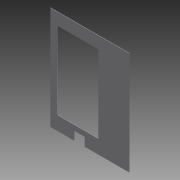
# Autodesk Inventor part: Right Side
Saved by Autodesk Inventor 2012 (Build 160160000, 160)
## iProperties
Created: 2012-04-20
Part Number: Right Side
Material: Default
Document SubType Name: Modeling
Designer: Puzzles
Density: 1 g/cm^3
Author: Puzzles
Autodesk Inventor part; units mm, degrees
ref_plane "YZ Plane" through (0, 0, 0) normal (1, 0, 0) x (0, 1, 0)
ref_plane "XZ Plane" through (0, 0, 0) normal (0, 1, 0) x (-1, 0, 0)
ref_plane "XY Plane" through (0, 0, 0) normal (0, 0, 1) x (1, 0, 0)
sketch "Sketch1" plane through (0, 0, 0) normal (0, 0, 1) x (1, 0, 0)
  line L0 (-292.1, 381) -> (292.1, 381)
  line L1 (292.1, 381) -> (292.1, -381)
  line L2 (292.1, -381) -> (-292.1, -381)
  line L3 (-292.1, -381) -> (-292.1, 381)
  point P0 (0, 0)
  point P1 (0, 381)
  point P2 (292.1, 0)
  dimension "d0" = 584.2
  dimension "d1" = 762
  constraints: 8 end point, 2 midpoint, 2 parallel, 1 horizontal, 1 horizontal alignment, 1 perpendicular, 1 vertical alignment
  measures "d0" distance of L0.start L0.end
  measures "d1" distance of L2.end L0.start
extrude "Extrusion1" add sketch "Sketch1" along normal blind 3
sketch "Sketch2" plane through (0, 0, 3) normal (0, 0, 1) x (1, 0, 0)
  line L0 (-292.1, -381) -> (-292.1, 381) projected
  line L1 (292.1, -381) -> (-292.1, -381) projected
  line L2 (-241.3, 292.1) -> (63.5, 292.1)
  line L3 (63.5, 292.1) -> (63.5, -279.4)
  line L4 (63.5, -279.4) -> (-241.3, -279.4)
  line L5 (-241.3, -279.4) -> (-241.3, 292.1)
  line L6 (-114.3, -381) -> (-38.1, -381)
  line L7 (-38.1, -381) -> (-38.1, -317.5)
  line L8 (-38.1, -317.5) -> (-114.3, -317.5)
  line L9 (-114.3, -317.5) -> (-114.3, -381)
  point P0 (0, 0)
  dimension "d4" = 101.6
  dimension "d5" = 50.8
  dimension "d6" = 571.5
  dimension "d7" = 304.8
  dimension "d8" = 177.8
  dimension "d9" = 76.2
  dimension "d10" = 63.5
  constraints: 16 end point, 4 parallel, 2 horizontal, 2 perpendicular, 1 point on line
  measures "d4" distance between parallel lines of L1 L4
  measures "d5" distance between parallel lines of L0 L5
  measures "d6" distance of L4.end L2.start
  measures "d7" distance of L2.start L2.end
  measures "d8" distance between parallel lines of L0 L9
  measures "d9" distance of L7.end L8.end
  measures "d10" distance between parallel lines of L1 L8
extrude "Extrusion2" cut sketch "Sketch2" against normal blind 3
body "Solid1"
